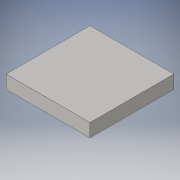
# Autodesk Inventor part: BindingPiece1
Saved by Autodesk Inventor 2016 (Build 200138000, 138)
## iProperties
Created: 2015-12-07
Part Number: BindingPiece1
Material: Generic
Document SubType Name: Modeling
Designer: Javier
Density: 1 g/cm^3
Appearance: Default
Author: Javier
Autodesk Inventor part; units mm, degrees
ref_plane "YZ Plane" through (0, 0, 0) normal (1, 0, 0) x (0, 1, 0)
ref_plane "XZ Plane" through (0, 0, 0) normal (0, 1, 0) x (-1, 0, 0)
ref_plane "XY Plane" through (0, 0, 0) normal (0, 0, 1) x (1, 0, 0)
sketch "Sketch1" plane through (0, 0, 0) normal (0, 0, 1) x (1, 0, 0)
  line L0 (-20, 3.175) -> (20, 3.175)
  line L1 (20, 3.175) -> (20, -3.175)
  line L2 (20, -3.175) -> (-20, -3.175)
  line L3 (-20, -3.175) -> (-20, 3.175)
  line L4 (0, 10.7485) -> (0, -11.1125)
  point P0 (0, 0)
  dimension "d5" = 40
  constraints: 10 end point, 2 parallel, 2 vertical, 1 horizontal, 1 perpendicular, 1 other
  measures "d5" distance of L0.start L0.end
extrude "Extrusion1" add sketch "Sketch1" along normal blind 40
sketch "Sketch2" plane through (0, 0, 0) normal (0, 1, 0) x (-1, 0, 0)
  circle A0 centre (0, 20) radius 7.9375
  circle A1 centre (0, 20) radius 9.525
  line L0 (20, 0) -> (-20, 0) projected
  point P0 (0, 0)
  dimension "d2" = 15.875
  dimension "d6" = 20
  constraints: 2 centre point, 1 coincident
  measures "d2" diameter of A0
  measures "d6" distance from line of A0.centre L0
extrude "Extrusion2" add sketch "Sketch2" against normal blind 10
body "Solid1"
